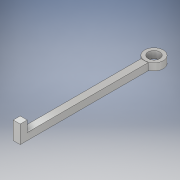
# Autodesk Inventor part: LegAnode
Saved by Autodesk Inventor 2019.3 (Build 233278000, 278)
## iProperties
Created: 2019-01-06
Part Number: LegAnode
Material: Aluminium 6061
Document SubType Name: Modeling
Designer: Jonas
Density: 2.7 g/cm^3
Appearance: Aluminium - poliert
Author: Jonas
Autodesk Inventor part; units mm, degrees
ref_plane "YZ Plane" through (0, 0, 0) normal (1, 0, 0) x (0, 1, 0)
ref_plane "XZ Plane" through (0, 0, 0) normal (0, 1, 0) x (-1, 0, 0)
ref_plane "XY Plane" through (0, 0, 0) normal (0, 0, 1) x (1, 0, 0)
sketch "Skizze1" plane through (0, 0, 0) normal (1, 0, 0) x (0, 1, 0)
  line L0 (1.7833, -0.9542) -> (0.85, -0.9542)
  line L1 (0.85, -0.9542) -> (0.85, -11.3542)
  line L2 (0.85, -11.3542) -> (0.25, -11.3542)
  line L3 (0.25, -11.3542) -> (0.25, -0.3542)
  line L4 (0.25, -0.3542) -> (1.7833, -0.3542)
  line L5 (1.7833, -0.3542) -> (1.7833, -0.9542)
  point P0 (0, 0)
  dimension "d0" = 0.6
  dimension "d1" = 0.6
  dimension "d2" = 11
  constraints: 12 end point, 5 perpendicular, 1 horizontal
  measures "d0" distance between parallel lines of L3 L1
  measures "d1" distance between parallel lines of L0 L4
  measures "d2" distance between parallel lines of L2 L4
extrude "Extrusion1" add sketch "Skizze1" along normal blind 0.6
sketch "Skizze4" plane through (0, 0.85, -0.9542) normal (0, 1, 0) x (1, 0, 0)
  line L0 (0, 10.4) -> (0.6, 10.4)
  line L1 (0, 10.4) -> (0.6, 10.4) projected
  circle A0 centre (0.3, 11.2) radius 0.8
  line L2 (0, 10.4) -> (0.6, 10.4) projected
  point P0 (0, -0.9542)
  dimension "d14" = 1.6
  constraints: 2 end point, 1 centre point, 1 tangent
  measures "d14" diameter of A0
extrude "Extrusion3" add sketch "Skizze4" against normal blind 0.6
sketch "Skizze6" plane through (0.3, 0.85, -12.1542) normal (0, 1, 0) x (1, 0, 0)
  circle A0 centre (0, 0) radius 0.5
  circle A1 centre (0, 0) radius 0.8 projected
  point P0 (-0.3, -12.1542)
  point P1 (0, -0.8)
  dimension "d15" = 1
  constraints: 1 centre point, 1 vertical alignment, 1 other
  measures "d15" diameter of A0
extrude "Extrusion5" cut sketch "Skizze6" against normal blind 0.6 contours A0
